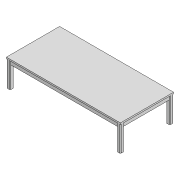
# Autodesk Inventor part: Table
Saved by Autodesk Inventor 2021 (Build 250183000, 183)
## iProperties
Created: 2021-04-29
Part Number: Table
Material: Generic
Document SubType Name: Modeling
Designer: Tran Duc Viet
Mass: 30036 g
Surface Area: 28090.7 cm^2
Volume: 30036 cm^3
Density: 1 g/cm^3
Appearance: Default
Author: Tran Duc Viet
Autodesk Inventor part; units mm, degrees
ref_plane "YZ Plane" through (0, 0, 0) normal (1, 0, 0) x (0, 1, 0)
ref_plane "XZ Plane" through (0, 0, 0) normal (0, 1, 0) x (-1, 0, 0)
ref_plane "XY Plane" through (0, 0, 0) normal (0, 0, 1) x (1, 0, 0)
sketch "Sketch1" plane through (0, 0, 0) normal (0, 1, 0) x (-1, 0, 0)
  line L0 (0, 0) -> (-50, 0)
  line L1 (-50, 0) -> (-50, -50)
  line L2 (-50, -50) -> (0, -50)
  line L3 (0, -50) -> (0, 0)
  line L4 (0, 0) -> (-1500, 0)
  line L5 (-1500, 0) -> (-1500, -700)
  line L6 (-1500, -700) -> (0, -700)
  line L7 (0, -700) -> (0, 0)
  line L8 (0, -700) -> (-50, -700)
  line L9 (-50, -700) -> (-50, -650)
  line L10 (-50, -650) -> (0, -650)
  line L11 (0, -650) -> (0, -700)
  line L12 (-1500, -700) -> (-1450, -700)
  line L13 (-1450, -700) -> (-1450, -650)
  line L14 (-1450, -650) -> (-1500, -650)
  line L15 (-1500, -650) -> (-1500, -700)
  line L16 (-1500, 0) -> (-1450, 0)
  line L17 (-1450, 0) -> (-1450, -50)
  line L18 (-1450, -50) -> (-1500, -50)
  line L19 (-1500, -50) -> (-1500, 0)
  point P0 (-1500, -50)
  point P1 (-1450, 0)
  point P2 (0, -650)
  dimension "d0" = 50
  dimension "d1" = 50
  dimension "d2" = 1500
  dimension "d3" = 700
  dimension "d4" = 50
  dimension "d5" = 50
  dimension "d6" = 50
  dimension "d7" = 50
  dimension "d8" = 50
  dimension "d9" = 50
  constraints: 40 end point, 10 parallel, 5 horizontal, 5 perpendicular
  measures "d0" distance of L2.end L1.end
  measures "d1" distance of L1.end L0.end
  measures "d2" distance of L6.end L5.end
  measures "d3" distance of L5.end L4.end
  measures "d4" distance of L9.end L10.end
  measures "d5" distance of L8.end L9.end
  measures "d6" distance of L14.end L13.end
  measures "d7" distance of L13.end L12.end
  measures "d8" distance of L17.end L18.end
  measures "d9" distance of L16.end L17.end
extrude "Extrusion1" add sketch "Sketch1" along normal blind 330 contours L3 L2 L1 L0 | L17 L18 L5 L4 | L7 L6 L9 L10 | L14 L13 L6 L5
sketch "Sketch2" plane through (0, 330, 0) normal (0, 1, 0) x (1, 0, 0)
  line L0 (50, 700) -> (0, 700) projected
  line L1 (0, 700) -> (1500, 700)
  line L2 (1500, 700) -> (1500, 0)
  line L3 (1500, 0) -> (0, 0)
  line L4 (0, 0) -> (0, 700)
  constraints: 8 end point, 2 parallel, 1 horizontal, 1 perpendicular
chamfer "Chamfer1" distance 10 angle 45 16 edges at (0, 165, -650) (50, 165, -650) (50, 165, -700) (0, 165, -700) (1450, 165, -650) (1450, 165, -700) (1500, 165, -700) (1500, 165, -650) (1450, 165, 0) (1500, 165, -50) (1500, 165, 0) (1450, 165, -50) (0, 165, -50) (0, 165, 0) (50, 165, 0) (50, 165, -50)
extrude "Extrusion2" add sketch "Sketch2" along normal blind 20
sketch "Sketch3" plane through (0, 330, 0) normal (0, -1, 0) x (1, 0, 0)
  line L0 (50, -10) -> (50, -40) projected
  line L1 (1450, -40) -> (1450, -10) projected
  line L2 (50, -10) -> (1450, -10)
  line L3 (1450, -10) -> (1450, -40)
  line L4 (1450, -40) -> (50, -40)
  line L5 (50, -40) -> (50, -10)
  line L6 (1490, -50) -> (1460, -50) projected
  line L7 (1460, -650) -> (1490, -650) projected
  line L8 (1460, -50) -> (1490, -50)
  line L9 (1490, -50) -> (1490, -650)
  line L10 (1490, -650) -> (1460, -650)
  line L11 (1460, -650) -> (1460, -50)
  line L12 (50, -660) -> (1450, -660)
  line L13 (1450, -660) -> (1450, -690)
  line L14 (1450, -690) -> (50, -690)
  line L15 (50, -690) -> (50, -660)
  line L16 (40, -50) -> (10, -50) projected
  line L17 (10, -50) -> (40, -50)
  line L18 (40, -50) -> (40, -650)
  line L19 (40, -650) -> (10, -650)
  line L20 (10, -650) -> (10, -50)
  point P0 (0, 0)
  constraints: 32 end point, 8 parallel, 4 horizontal, 4 perpendicular
extrude "Extrusion3" add sketch "Sketch3" along normal blind 50
body "Solid1"
